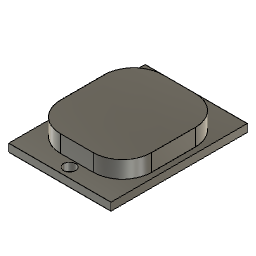
trackball-holder-mk4 v2 (Autodesk Fusion 360 archive; units mm, degrees)
design "PMW3360"
Autodesk Fusion 360 part; units mm, degrees
sketch "Sketch1" plane through (0, 0, 0) normal (0, 0, 1) x (1, 0, 0)
  line L0 (0, 0) -> (0, 28) construction
  line L1 (0, 28) -> (21, 28) construction
  line L2 (21, 28) -> (0, 28) construction
  line L3 (0, 28) -> (0, 0) construction
  line L4 (0, 0) -> (21, 0) construction
  line L5 (21, 0) -> (21, 28) construction
  line L6 (10.5, 0) -> (10.5, 28) construction
  line L7 (10.5, 0) -> (10.5, 2) construction
  line L8 (10.5, 28) -> (10.5, 26) construction
  circle A0 centre (10.5, 26) radius 1.25 construction
  circle A1 centre (10.5, 2) radius 1.25 construction
  line L9 (21, 28) -> (0, 28)
  line L10 (0, 28) -> (0, 0)
  line L11 (0, 0) -> (21, 0)
  line L12 (21, 0) -> (21, 28)
  circle A2 centre (10.5, 2) radius 1.25
  circle A3 centre (10.5, 26) radius 1.25
  dimension "d38" = 28
  dimension "d39" = 21
  dimension "d40" = 2
  dimension "d41" = 2
  dimension "d42" = 2.5
  dimension "d43" = 2.5
  constraint coincident L0.start L3.end
  constraint vertical L0
  constraint perpendicular L0 L1
  constraint horizontal L2
  constraint vertical L3
  constraint horizontal L4
  constraint vertical L5
  constraint midpoint L4 L6.start
  constraint midpoint L2 L6.end
  constraint perpendicular L4 L7
  constraint perpendicular L1 L8
  constraint coincident L8.end A0.centre
  constraint coincident L7.end A1.centre
  constraint horizontal L9
  constraint vertical L10
  constraint horizontal L11
  constraint vertical L12
  constraint concentric A1 A2
  constraint concentric A0 A3
  measures "d38" distance of L0.start L0.end
  measures "d39" distance of L0.end L1.end
  measures "d40" distance of L6.start L7.end
  measures "d41" distance of L6.end L8.end
  measures "d42" diameter of A0
  measures "d43" diameter of A1
extrude "Extrude1" add sketch "Sketch1" along normal blind 1.6
sketch "Sketch2" plane through (0, 0, 1.6) normal (0, 0, 1) x (-1, 0, 0)
  circle A0 centre (-10.5, -26) radius 1.25
  circle A1 centre (-10.5, -2) radius 1.25
  line L0 (-21, 0) -> (-21, -28)
  line L1 (-21, -28) -> (0, -28)
  line L2 (0, -28) -> (0, 0)
  line L3 (0, 0) -> (-21, 0)
  line L4 (0, -14) -> (-21, -14) construction
  line L5 (-10.5, -28) -> (-10.5, 0) construction
  line L6 (-10.5, -14) -> (-10.5, -24.5) construction
  line L7 (-10.5, -24.5) -> (-19.85, -24.5) construction
  line L8 (-10.5, -14) -> (-10.5, -3.5) construction
  line L9 (-10.5, -3.5) -> (-1.15, -3.5) construction
  line L10 (-1.15, -3.5) -> (-19.85, -3.5) construction
  line L11 (-19.85, -3.5) -> (-19.85, -24.5) construction
  line L12 (-19.85, -24.5) -> (-1.15, -24.5) construction
  line L13 (-1.15, -24.5) -> (-1.15, -3.5) construction
  line L14 (-1.15, -3.5) -> (-19.85, -3.5)
  line L15 (-19.85, -3.5) -> (-19.85, -24.5)
  line L16 (-19.85, -24.5) -> (-1.15, -24.5)
  line L17 (-1.15, -24.5) -> (-1.15, -3.5)
  dimension "d46" = 10.5
  dimension "d47" = 9.35
  dimension "d48" = 10.5
  dimension "d49" = 9.35
  constraint midpoint L2 L4.start
  constraint midpoint L0 L4.end
  constraint midpoint L1 L5.start
  constraint midpoint L3 L5.end
  constraint midpoint L5 L6.start
  constraint perpendicular L4 L6
  constraint perpendicular L6 L7
  constraint perpendicular L7 L8
  constraint perpendicular L5 L9
  constraint horizontal L10
  constraint vertical L11
  constraint horizontal L12
  constraint vertical L13
  constraint horizontal L14
  constraint vertical L15
  constraint horizontal L16
  constraint vertical L17
  measures "d46" distance of L6.start L6.end
  measures "d47" distance of L6.end L7.end
  measures "d48" distance of L6.start L8.end
  measures "d49" distance of L8.end L9.end
extrude "Extrude2" add sketch "Sketch2" along normal blind 3.5 contours L14 L15 L16 L17
fillet "Fillet1" radius 6 4 edges at (19.85, 3.5, 3.35) (1.15, 3.5, 3.35) (1.15, 24.5, 3.35) (19.85, 24.5, 3.35)

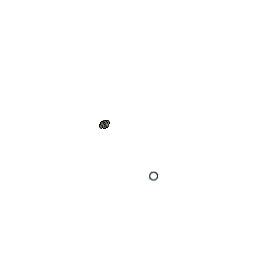
design "Mini-Bearing"
Autodesk Fusion 360 part; units mm, degrees
sketch "Sketch1" plane through (0, 0, 0) normal (0, 0, 1) x (1, 0, 0)
  circle A0 centre (0, 0) radius 3.5
  circle A1 centre (0, 0) radius 1.95
  dimension "d85" = 7
  dimension "d86" = 3.9
  constraint coincident A0.centre A1.centre
  measures "d85" diameter of A0
  measures "d86" diameter of A1
extrude "Extrude1" add sketch "Sketch1" along normal blind 2.5
sketch "Sketch2" plane through (0, 0, 0) normal (0, 0, 1) x (1, 0, 0)
  circle A0 centre (0, 0) radius 2
  constraint coincident A0.centre origin
extrude "Extrude2" add sketch "Sketch2" against normal blind 3
extrude "Extrude3" add 1 faces at (-0.325, 0.3213, 0) along direction (0, 0, 1) blind 5.5
move_body "Move1" bodies 1 to x (1, 0, 0) y (0, 1, 0) z (0, 0, 1) at (-1.4953, -0.1188, 0)
sketch "sketch 496" plane through (73.8903, -150.6507, -43.9901) normal (-0.866025, 0, 0.5) x (-0.5, 0, -0.866025)
  line L0 (-95.4904, -88.9756) -> (-91.7882, -86.9923)
  line L1 (-95.4904, -88.9756) -> (-91.7882, -86.9923)
  line L2 (-91.7882, -86.9923) -> (-92.5153, -85.635)
  arc A0 (-92.5153, -85.635) -> (-96.5133, -87.0663) centre (-93.3717, -89.5423) ccw
  line L3 (-95.4904, -88.9756) -> (-96.5133, -87.0663)
  line L4 (-89.6444, -90.994) -> (-90.3715, -89.6367)
  line L5 (-90.3715, -89.6367) -> (-94.0738, -91.6201)
  line L6 (-90.3715, -89.6367) -> (-94.0738, -91.6201)
  line L7 (-93.0509, -93.5294) -> (-94.0738, -91.6201)
  arc A1 (-93.0509, -93.5294) -> (-89.6444, -90.994) centre (-93.3717, -89.5423) ccw
  arc A2 (-93.0509, -93.5294) -> (-89.6444, -90.994) centre (-93.3717, -89.5423) ccw
extrude "Extrude4" cut sketch "sketch 496" against normal blind 5
move_body "Move2" bodies 1 to x (1, 0, 0) y (0, 0, 1) z (0, -1, 0) at (0, 2.3812, 2.6188)
move_body "Move3" bodies 1 to x (1, 0, 0) y (0, 1, 0) z (0, 0, 1) at (1.5, -1.1, -2.5)
ref_plane "WorkPlane1" through (1.9547, -2.6103, 0) normal (1, 0, 0) x (0, 0, -1)
ref_plane "WorkPlane2" through (0.0047, -2.6103, 0) normal (1, 0, 0) x (0, 0, -1)
